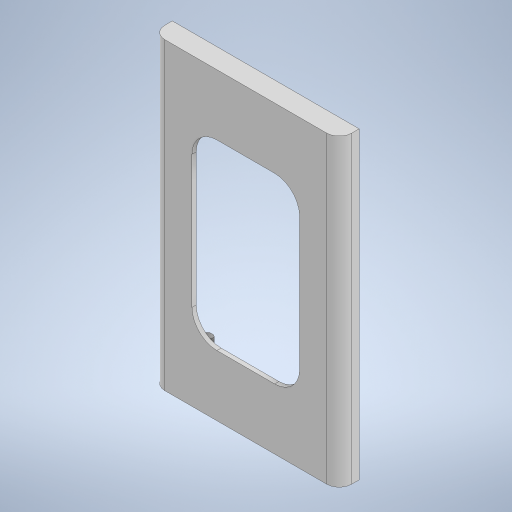
# Autodesk Inventor part: 스위치 커버
Saved by Autodesk Inventor 2023 (Build 270158000, 158)
## iProperties
Created: 2022-06-24
Part Number: 스위치 커버
Material: 일반
Document SubType Name: Modeling
Designer: user
Density: 1 g/cm^3
Appearance: 기본값
Author: user
Autodesk Inventor part; units mm, degrees
ref_plane "YZ Plane" through (0, 0, 0) normal (1, 0, 0) x (0, 1, 0)
ref_plane "XZ Plane" through (0, 0, 0) normal (0, 1, 0) x (-1, 0, 0)
ref_plane "XY Plane" through (0, 0, 0) normal (0, 0, 1) x (1, 0, 0)
sketch "스케치1" plane through (0, 0, 0) normal (0, 0, 1) x (1, 0, 0)
  line L0 (-37.5, 61) -> (37.5, 61)
  line L1 (37.5, 61) -> (37.5, -61)
  line L2 (37.5, -61) -> (-37.5, -61)
  line L3 (-37.5, -61) -> (-37.5, 61)
  line L4 (-37.5, 61) -> (37.5, -61) construction
  line L5 (37.5, 61) -> (-37.5, -61) construction
  line L6 (-21.6, 36.6) -> (21.6, 36.6)
  line L7 (21.6, 36.6) -> (21.6, -36.6)
  line L8 (21.6, -36.6) -> (-21.6, -36.6)
  line L9 (-21.6, -36.6) -> (-21.6, 36.6)
  line L10 (-21.6, 36.6) -> (21.6, -36.6) construction
  line L11 (21.6, 36.6) -> (-21.6, -36.6) construction
  point P0 (0, 0)
  dimension "d0" = 75
  dimension "d1" = 122
  dimension "d2" = 43.2
  dimension "d3" = 73.2
  constraints: 24 end point, 4 midpoint, 4 parallel, 2 horizontal, 2 perpendicular
  measures "d0" distance of L1.end L2.end
  measures "d1" distance of L0.end L1.end
  measures "d2" distance of L7.end L8.end
  measures "d3" distance of L6.end L7.end
extrude "돌출1" add sketch "스케치1" along normal blind 8
fillet "모깎기1" radius 5 2 edges at (37.5, 0, 8) (-37.5, 0, 8)
shell "쉘1" thickness 1.7 removed faces 1 at (32.2, -12.2, 0)
sketch "스케치2" plane through (32.5, 59.3, 6.3) normal (0, 0, -1) x (-1, 0, 0)
  line L0 (6.4857, -104.5153) -> (58.5143, -104.5153)
  line L1 (58.5143, -104.5153) -> (58.5143, -14.0847)
  line L2 (58.5143, -14.0847) -> (6.4857, -14.0847)
  line L3 (6.4857, -14.0847) -> (6.4857, -104.5153)
  line L4 (6.4857, -104.5153) -> (58.5143, -14.0847) construction
  line L5 (58.5143, -104.5153) -> (6.4857, -14.0847) construction
  point P0 (32.5, -59.3)
  constraints: 12 end point, 2 midpoint, 2 parallel, 1 horizontal, 1 perpendicular
extrude "돌출2" cut sketch "스케치2" along normal blind 8
sketch "스케치3" plane through (32.5, 59.3, 6.3) normal (0, 0, -1) x (-1, 0, 0)
  line L0 (53.65, -14.6) -> (60.65, -14.6)
  line L1 (60.65, -14.6) -> (60.65, -19.3)
  line L2 (60.65, -19.3) -> (53.65, -19.3)
  line L3 (53.65, -19.3) -> (53.65, -14.6)
  line L4 (53.65, -14.6) -> (60.65, -19.3) construction
  line L5 (60.65, -14.6) -> (53.65, -19.3) construction
  line L6 (53.65, -14.6) -> (57.15, -14.6)
  line L7 (57.15, -14.6) -> (57.15, -19.3)
  line L8 (57.15, -19.3) -> (53.65, -19.3)
  line L9 (53.65, -19.3) -> (53.65, -14.6)
  point P0 (32.5, -59.3)
  point P1 (57.15, -16.95)
  point P2 (57.15, -14.6)
  dimension "d10" = 40
  dimension "d11" = 4.7
  dimension "d12" = 7
  dimension "d13" = 21.15
  constraints: 20 end point, 4 parallel, 3 midpoint, 2 horizontal, 2 perpendicular
  measures "d10" distance from line of point (32.5, -59.3) L2
  measures "d11" distance of L0.end L1.end
  measures "d12" distance of L0.start L0.end
  measures "d13" distance from line of point (32.5, -59.3) L3
extrude "돌출3" add sketch "스케치3" along normal blind 6.5 contours L0 L7 L2 L3
chamfer "모따기1" distance 2 angle 45 1 edges at (-24.65, 42.35, -0.2)
sketch "스케치4" plane through (-24.65, 40, 6.3) normal (0, -1, 0) x (1, 0, 0)
  line L0 (2, -6.5) -> (3.5, -6.5) projected
  line L1 (4.4338, -4.6675) -> (3.5, -4)
  line L2 (3.5, 0) -> (3.5, -6.5) projected
  line L3 (4.4338, -4.6675) -> (4.4338, -5.8892)
  line L4 (4.4338, -5.8892) -> (3.5, -6.5)
  point P0 (24.65, -6.3)
  dimension "d19" = 4
  constraints: 6 end point, 1 point on line, 1 vertical
  measures "d19" distance of L2.start L1.end
extrude "돌출4" add sketch "스케치4" against normal blind 4.7
mirror "미러1" about plane through (0, 0, 0) normal (0, 1, 0) of "돌출4", "돌출3", "모따기1"
mirror "미러2" about plane through (0, 0, 0) normal (1, 0, 0) of "돌출4", "돌출3", "모따기1", "미러1"
fillet "모깎기2" radius 10 4 edges at (21.6, -36.6, 7.15) (-21.6, -36.6, 7.15) (21.6, 36.6, 7.15) (-21.6, 36.6, 7.15)
